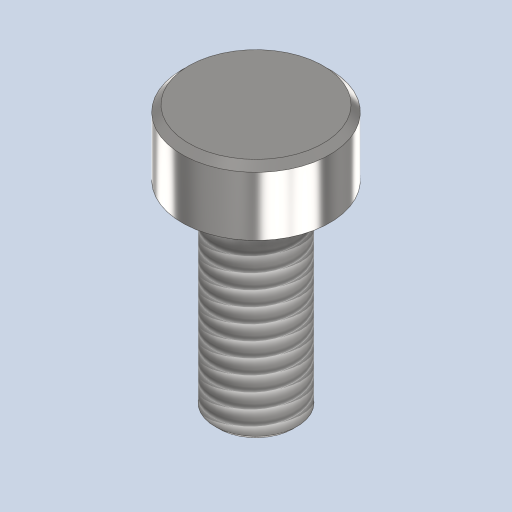
# Autodesk Inventor part: CSH-316L-M2-5
Saved by Autodesk Inventor 2023 (Build 270158000, 158)
## iProperties
Created: 2024-11-11
Part Number: CSH-316L-M2-5
Material: ステンレス鋼
Document SubType Name: Modeling
Designer: kiyo
Density: 8 g/cm^3
Appearance: 半つや出し
Mass: 0.551073 g
Surface Area: 1.11996 cm^2
Volume: 0.0688841 cm^3
Author: kiyo
Autodesk Inventor part; units mm, degrees
ref_plane "YZ Plane" through (0, 0, 0) normal (1, 0, 0) x (0, 1, 0)
ref_plane "XZ Plane" through (0, 0, 0) normal (0, 1, 0) x (-1, 0, 0)
ref_plane "XY Plane" through (0, 0, 0) normal (0, 0, 1) x (1, 0, 0)
sketch "スケッチ1" plane through (0, 0, 0) normal (1, 0, 0) x (0, 1, 0)
  line L0 (0, 0) -> (1.25, 0)
  line L1 (1.25, 0) -> (1.25, -6)
  line L2 (1.25, -6) -> (0, -6)
  line L3 (0, -6) -> (0, 0)
  line L4 (0, -6) -> (2.25, -6)
  line L5 (2.25, -6) -> (2.25, -8)
  line L6 (2.25, -8) -> (0, -8)
  line L7 (0, -8) -> (0, -6)
  line L8 (2.25, -7.8) -> (2.05, -8)
  line L9 (1.25, -0.12) -> (1.13, 0)
  point P0 (2.25, -7)
  dimension "d0" = 45
  dimension "d1" = 2.25
  dimension "d2" = 2
  dimension "d3" = 6
  dimension "d7" = 1.25
  dimension "d10" = 45
  dimension "d11" = 0.2
  dimension "d12" = 0.12
  constraints: 20 end point, 4 parallel, 4 point on line, 2 horizontal, 2 perpendicular, 1 midpoint
  measures "d0" angle of L8 L5
  measures "d1" distance from line of L7 point (2.25, -7)
  measures "d2" distance of L4.end L5.end
  measures "d3" distance of L0.end L1.end
  measures "d7" distance between parallel lines of L3 L1
  measures "d10" angle of L9 L1
  measures "d11" distance from line of L8.start L6
  measures "d12" distance from line of L9.start L0
revolve "回転1" add sketch "スケッチ1" angle 360 about axis through (0, 0, -6) along (0, 0, 1) contours L0 L9 L1 L2 L3 | L2 L4 L5 L8 L6 L7
thread "ねじ2" size "M2.5x0.45" class "6g" standard "ANSI Metric M Profile" length 30
